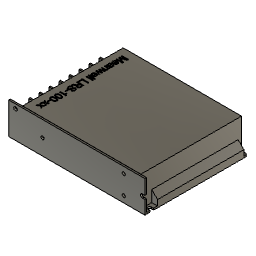
Meanwell LRS-100-xx v3 (Autodesk Fusion 360 design; units mm, degrees)
Autodesk Fusion 360 part; units mm, degrees
note: some values were not read from the file. Set by a fixed rule: which sketch regions a step uses.
sketch "Sketch1" plane through (0, 0, 0) normal (0, 0, 1) x (1, 0, 0)
  line L0 (0, 0) -> (129, 0)
  line L1 (129, 97) -> (0, 97)
  line L2 (0, 97) -> (0, 0)
  line L3 (11.5, 97) -> (11.5, 1.7)
  line L4 (11.5, 1.7) -> (123.5, 1.7)
  line L5 (123.5, 1.7) -> (123.5, 97)
  circle A0 centre (4.5, 91.5) radius 1.75
  line L6 (127, 8.25) -> (129, 8.25)
  line L7 (127, 4.75) -> (129, 4.75)
  line L8 (129, 0) -> (129, 4.75)
  line L9 (129, 8.25) -> (129, 97)
  arc A1 (127, 8.25) -> (127, 4.75) centre (127, 6.5) ccw
  line L10 (129, 1.6) -> (0, 1.6)
  circle A2 centre (78, 34) radius 1.5
  line L11 (78, 34) -> (78, 67) construction
  circle A3 centre (78, 67) radius 1.5
  dimension "d1" = 129
  dimension "d2" = 97
  dimension "d3" = 3.5
  dimension "d4" = 4.5
  dimension "d5" = 91.5
  dimension "d6" = 3.5
  dimension "d7" = 6.5
  dimension "d8" = 127
  dimension "d9" = 11.5
  dimension "d10" = 1.6
  dimension "d11" = 0.1
  dimension "d12" = 123.5
  dimension "d62" = 3
  dimension "d63" = 3
  dimension "d64" = 78
  dimension "d65" = 34
  dimension "d66" = 33
  constraint horizontal L0
  constraint vertical L8
  constraint horizontal L1
  constraint vertical L2
  constraint coincident L0.start L2.end
  constraint coincident L1 L3.start
  constraint perpendicular L1 L3
  constraint perpendicular L3 L4
  constraint coincident L1 L5.end
  constraint perpendicular L1 L5
  constraint coincident L6.end L8
  constraint tangent L6 A1
  constraint horizontal L6
  constraint horizontal L7
  constraint tangent L7 A1
  constraint collinear L8 L9
  constraint coincident L8 L10.start
  constraint coincident L2 L10.end
  constraint perpendicular L2 L10
  constraint coincident A2.centre L11.start
  constraint parallel L5 L11
  constraint coincident L11.end A3.centre
  measures "d1" distance of L1.start L1.end
  measures "d2" distance of L0.start L1.end
  measures "d3" diameter of A0
  measures "d4" distance of L2 A0.centre
  measures "d5" distance of L0 A0.centre
  measures "d6" diameter of A1
  measures "d7" distance of L0 A1.centre
  measures "d8" distance of L2 A1.centre
  measures "d9" distance of L2 L3
  measures "d10" distance of L0 L10
  measures "d11" distance of L4 L10
  measures "d12" distance of L2 L5
  measures "d62" diameter of A2
  measures "d63" diameter of A3
  measures "d64" distance of L2 L11
  measures "d65" distance of L0 A2.centre
  measures "d66" distance of A2.centre L11.end
extrude "Extrude1" add sketch "Sketch1" along normal blind 30 contours L0 L2 L8 L10
extrude "Extrude2" add sketch "Sketch1" along normal blind 1.6 contours L1 L2 L3 L4 L5 L6 L7 L8 L9 A1 L10 | L1 L3 L4 L5
extrude "Extrude3" add sketch "Sketch1" along normal blind 28.4 from surface at 1.6 contours L1 L3 L4 L5 | A2 | A3
sketch "Sketch2" plane through (0, 0, 1.6) normal (0, 0, 1) x (-1, 0, 0)
  line L0 (-123.5, -97) -> (-123.5, -1.7)
  line L1 (-123.5, -1.7) -> (-11.5, -1.7)
  line L2 (-11.5, -1.7) -> (-11.5, -97)
  line L3 (-11.5, -97) -> (0, -97)
  line L4 (0, -97) -> (0, -1.6)
  line L5 (0, -1.6) -> (-129, -1.6)
  line L6 (-129, -1.6) -> (-129, -4.75)
  line L7 (-129, -4.75) -> (-127, -4.75)
  arc A0 (-127, -8.25) -> (-127, -4.75) centre (-127, -6.5) ccw
  line L8 (-127, -8.25) -> (-129, -8.25)
  line L9 (-129, -8.25) -> (-129, -97)
  line L10 (-129, -97) -> (-123.5, -97)
  circle A1 centre (-4.5, -91.5) radius 1.75
  line L11 (0, -87) -> (-11.5, -87)
  line L12 (-11.5, -19) -> (0, -19)
  circle A2 centre (-5.75, -81.55) radius 3
  circle A3 centre (-5.75, -72.05) radius 3
  circle A4 centre (-5.75, -62.55) radius 3
  circle A5 centre (-5.75, -53.05) radius 3
  circle A6 centre (-5.75, -43.55) radius 3
  circle A7 centre (-5.75, -34.05) radius 3
  circle A8 centre (-5.75, -24.55) radius 3
  line L13 (0, -85.6) -> (-11.5, -85.6)
  line L14 (0, -77.5) -> (-11.5, -77.5)
  line L15 (0, -76.1) -> (-11.5, -76.1)
  line L16 (0, -68) -> (-11.5, -68)
  line L17 (0, -66.6) -> (-11.5, -66.6)
  line L18 (0, -58.5) -> (-11.5, -58.5)
  line L19 (0, -57.1) -> (-11.5, -57.1)
  line L20 (0, -49) -> (-11.5, -49)
  line L21 (0, -47.6) -> (-11.5, -47.6)
  line L22 (0, -39.5) -> (-11.5, -39.5)
  line L23 (0, -38.1) -> (-11.5, -38.1)
  line L24 (0, -30) -> (-11.5, -30)
  line L25 (0, -28.6) -> (-11.5, -28.6)
  line L26 (0, -20.5) -> (-11.5, -20.5)
  line L27 (0, -19.1) -> (-11.5, -19.1)
  line L28 (-129, -97) -> (0, -97)
  circle A9 centre (-4.4499, -10.6037) radius 3.25
  circle A10 centre (-10.3253, -10.679) radius 1.5
  line L29 (0, -1.6) -> (0, -19.1)
  line L30 (-11.5, -1.7) -> (-11.5, -1.6)
  dimension "d19" = 6
  dimension "d22" = 0
  dimension "d23" = 9.5
  dimension "d25" = 68
  dimension "d26" = 1.4
  dimension "d29" = 0
  dimension "d30" = 9.5
  dimension "d31" = 5.45
  dimension "d32" = 10
  dimension "d33" = 6.5
  dimension "d34" = 3
  constraint coincident L4 L11.start
  constraint coincident L2 L11.end
  constraint perpendicular L2 L11
  constraint coincident L2 L12.start
  constraint coincident L4 L12.end
  constraint perpendicular L4 L12
  constraint coincident L4 L13.start
  constraint coincident L2 L13.end
  constraint perpendicular L2 L13
  constraint coincident L4.end L5.start
  constraint coincident L1.end L2.start
  constraint coincident L5 L30.end
  constraint perpendicular L5 L30
  measures "d19" diameter of A2
  measures "d25" distance of L11 L12
  measures "d26" distance of L11 L13
  measures "d31" distance of L11 A2.centre
  measures "d32" distance of L11 L28
  measures "d33" diameter of A9
  measures "d34" diameter of A10
extrude "Extrude4" add sketch "Sketch2" along normal blind 12.3 contours L2 L4 L13 L14 | L2 L4 L15 L16 | L2 L4 L25 L26 | L2 L4 L17 L18 | L2 L4 L23 L24 | L2 L4 L19 L20 | L2 L4 L21 L22 | A2 | A3 | A4 | A5 | A6 | A7 | A8
extrude "Extrude5" add sketch "Sketch2" along normal blind 20 contours L2 L4 L11 L13 | L2 L4 L14 L15 | L2 L4 L26 L27 | L2 L4 L16 L17 | L2 L4 L24 L25 | L2 L4 L18 L19 | L2 L4 L22 L23 | L2 L4 L20 L21
extrude "Extrude6" add sketch "Sketch2" along normal blind 15.328 contours A2 | A3 | A4 | A5 | A6 | A7 | A8
extrude "Extrude7" add sketch "Sketch2" along normal blind 4.4 contours L2 L4 L5 L12 A10 L29 L30 | L2 A10 | A9 picked at (-10.1005, -10.5525)
extrude "Extrude8" add sketch "Sketch2" along normal blind 12.4 contours L2 A10 | L2 A10 | A9
sketch "Sketch3" plane through (0, 0, 0) normal (0, -1, 0) x (1, 0, 0)
  line L0 (0, 0) -> (129, 0)
  line L1 (129, 0) -> (129, 30)
  line L2 (129, 30) -> (0, 30)
  line L3 (0, 30) -> (0, 0)
  circle A0 centre (6.5, 26) radius 1.75
  line L4 (126.5, 16.25) -> (129, 16.25)
  line L5 (126.5, 12.75) -> (129, 12.75)
  arc A1 (126.5, 16.25) -> (126.5, 12.75) centre (126.5, 14.5) ccw
  line L6 (129, 16.25) -> (129, 12.75)
  circle A2 centre (32, 15) radius 1.5
  circle A3 centre (109, 24) radius 1.5
  circle A4 centre (109, 6) radius 1.5
  line L7 (129, 0) -> (129, 6.8)
  line L8 (129, 6.8) -> (123.5, 12.3)
  line L9 (123.5, 0) -> (123.5, 30) construction
  line L10 (123.5, 12.3) -> (123.5, 0)
  point P0 (123.5, 0)
  dimension "d45" = 3.5
  dimension "d46" = 3.5
  dimension "d47" = 14.5
  dimension "d48" = 126.5
  dimension "d49" = 26
  dimension "d50" = 6.5
  dimension "d51" = 3
  dimension "d52" = 32
  dimension "d53" = 15
  dimension "d54" = 77
  dimension "d55" = 3
  dimension "d56" = 3
  dimension "d57" = 77
  dimension "d58" = 6
  dimension "d59" = 18
  dimension "d68" = 6.8
  dimension "d69" = 45
  constraint coincident L1 L4.end
  constraint coincident L1 L5.end
  constraint horizontal L4
  constraint horizontal L5
  constraint tangent L4 A1
  constraint tangent L5 A1
  constraint coincident L0.end L1.start
  constraint coincident L1 L7.end
  constraint perpendicular L0 L7
  constraint coincident P0 L9.start
  constraint coincident L2 L9.end
  constraint perpendicular L2 L9
  constraint coincident L8.end L9
  measures "d45" diameter of A0
  measures "d46" diameter of A1
  measures "d47" distance of L0 A1.centre
  measures "d48" distance of L3 A1.centre
  measures "d49" distance of L0 A0.centre
  measures "d50" distance of L3 A0.centre
  measures "d51" diameter of A2
  measures "d52" distance of L3 A2.centre
  measures "d53" distance of L0 A2.centre
  measures "d54" horizontal distance of A2.centre A4.centre
  measures "d55" diameter of A4
  measures "d56" diameter of A3
  measures "d57" horizontal distance of A2.centre A3.centre
  measures "d58" distance of L0 A4.centre
  measures "d59" distance of A3.centre A4.centre
  measures "d68" distance of L0.end L7.end
  measures "d69" angle of L8 L9
extrude "Extrude10" add sketch "Sketch3" against normal blind 81.8 from surface at -12 contours L0 L1 L7 L8 L10
extrude "Extrude9" cut sketch "Sketch3" against normal blind 1.6 contours L1 L4 L5 A1 L6 | A0 | A2 | A3 | A4
fillet "Fillet1" radius 1 2 edges at (129, 97, 0.8) (0, 97, 0.8)
sketch "Sketch4" plane through (0, 0, 30) normal (0, 0, 1) x (-1, 0, 0)
  line L0 (-123.5, -1.7) -> (-123.5, -97)
  line L1 (-123.5, -97) -> (-11.5, -97)
  line L2 (-11.5, -97) -> (-11.5, -1.7)
  line L3 (-11.5, -1.7) -> (-123.5, -1.7)
  line L4 (-11.5, -97) -> (-11.5, -1.7) construction
  line L5 (-11.5, -1.7) -> (-23.4855, -1.7) construction
  line L6 (-23.4855, -1.7) -> (-23.4855, -97) construction
  line L7 (-23.4855, -97) -> (-11.5, -97) construction
  dimension "d75" = 6
  text T0 "Meanwell LRS-100-xx" font "Arial" height 6 align centre top in box 95.3 x 11.9855 at (-11.5, -97) x (0, 1) y (-1, 0) spacing 1
  constraint coincident L3
  constraint coincident L1.end
extrude "Extrude11" cut sketch "Sketch4" against normal blind 0.4 text T0
equation "d5 = 85 mm + 6.5 mm"
equation "d8 = 122.5 mm + 4.5 mm"
equation "d17 = 30 mm - 1.6 mm"
equation "d31 = ( ( 9.5 / 2 ) * 1 mm ) + 0.7 mm"
equation "d35 = 13.9 mm - 1.6 mm"
equation "d41 = 6 mm - 1.6 mm"
equation "d43 = 14 mm - 1.6 mm"
named bodies: "LRS-100-xx"
